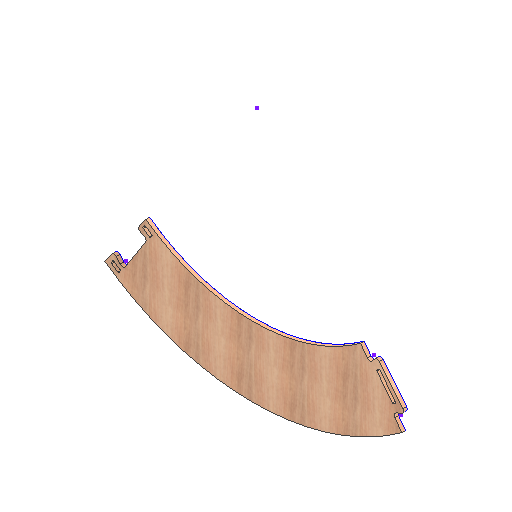
# Autodesk Inventor part: Platform C3
Saved by Autodesk Inventor 2021 (Build 250183000, 183)
## iProperties
Created: 2020-05-09
Part Number: Platform C3
Material: Wood (Birch)
Document SubType Name: Modeling
Designer: Dan Wikman
Density: 0.55 g/cm^3
Appearance: Birch - Natural Polished
Mass: 4368.22 g
Surface Area: 9555.55 cm^2
Volume: 7942.21 cm^3
Autodesk Inventor part; units mm, degrees
ref_plane "YZ Plane" through (0, 0, 0) normal (1, 0, 0) x (0, 1, 0)
ref_plane "XZ Plane" through (0, 0, 0) normal (0, 1, 0) x (-1, 0, 0)
ref_plane "XY Plane" through (0, 0, 0) normal (0, 0, 1) x (1, 0, 0)
sketch "CONTOURS" plane through (0, 0, 0) normal (0, 0, 1) x (1, 0, 0)
  line L0 (1187.1814, 538.0239) -> (1154.7956, 493.4487)
  arc A0 (1154.7956, 493.4487) -> (1161.7152, 471.2473) centre (1166.5264, 484.9258) ccw
  line L1 (1161.7152, 471.2473) -> (1177.6489, 465.6429)
  arc A1 (1185.5445, 442.6399) -> (1177.6489, 465.6429) centre (1172.5058, 451.021) ccw
  line L2 (1185.5445, 442.6399) -> (1088.242, 291.2628)
  arc A2 (1063.4384, 289.5524) -> (1088.242, 291.2628) centre (1075.2033, 299.6438) ccw
  line L3 (1063.4384, 289.5524) -> (1044.645, 311.4625)
  arc A3 (1044.645, 311.4625) -> (1021.9083, 310.545) centre (1033.6391, 302.0221) ccw
  line L4 (1021.9083, 310.545) -> (988.51, 264.5762)
  arc A4 (988.51, 264.5762) -> (2420.2584, 264.576) centre (1704.3843, 1251.0758) ccw
  line L5 (2420.2584, 264.576) -> (2386.86, 310.545)
  arc A5 (2393.4378, 333.9632) -> (2386.86, 310.545) centre (2399.3997, 319.6557) ccw
  line L6 (2393.4378, 333.9632) -> (2420.083, 345.0663)
  arc A6 (2420.083, 345.0663) -> (2425.7316, 367.6284) centre (2414.5057, 358.4507) ccw
  line L7 (2425.7316, 367.6284) -> (2311.8314, 506.9467)
  arc A7 (2311.8314, 506.9467) -> (2289.0833, 506.5717) centre (2300.6056, 497.769) ccw
  line L8 (2289.0833, 506.5717) -> (2278.8294, 493.1497)
  arc A8 (2253.9726, 493.4487) -> (2278.8294, 493.1497) centre (2266.5124, 502.5594) ccw
  line L9 (2253.9726, 493.4487) -> (2221.5869, 538.0239)
  arc A9 (1187.1814, 538.0239) -> (2221.5869, 538.0239) centre (1704.3841, 1250.9821) ccw
  constraints: 20 end point, 20 point on circle, 10 centre point
sketch "HOLES" plane through (0, 0, 0) normal (0, 0, 1) x (1, 0, 0)
  arc A0 (1185.5871, 509.2559) -> (1180.0259, 508.2196) centre (1183.3247, 505.9572) ccw
  line L0 (1185.5871, 509.2559) -> (1215.2756, 488.8945)
  arc A1 (1216.312, 483.3334) -> (1215.2756, 488.8945) centre (1213.0133, 485.5957) ccw
  line L1 (1216.312, 483.3334) -> (1210.0905, 474.2619)
  arc A2 (1204.5293, 473.2255) -> (1210.0905, 474.2619) centre (1206.7917, 476.5242) ccw
  line L2 (1204.5293, 473.2255) -> (1174.8407, 493.5869)
  arc A3 (1173.8044, 499.148) -> (1174.8407, 493.5869) centre (1177.1031, 496.8857) ccw
  line L3 (2383.598, 366.9908) -> (2380.4297, 364.5491)
  arc A4 (2374.8197, 365.2756) -> (2380.4297, 364.5491) centre (2377.988, 367.7173) ccw
  line L4 (2374.8197, 365.2756) -> (2300.3458, 461.907)
  arc A5 (2301.0723, 467.5171) -> (2300.3458, 461.907) centre (2303.5141, 464.3488) ccw
  line L5 (2301.0723, 467.5171) -> (2309.785, 474.2319)
  arc A6 (2315.395, 473.5054) -> (2309.785, 474.2319) centre (2312.2268, 471.0637) ccw
  line L6 (2315.395, 473.5054) -> (2389.8689, 376.874)
  arc A7 (2389.1424, 371.2639) -> (2389.8689, 376.874) centre (2386.7006, 374.4322) ccw
  line L7 (2389.1424, 371.2639) -> (2383.598, 366.9908)
  line L8 (1063.375, 260.339) -> (1057.1535, 251.2675)
  arc A8 (1051.5924, 250.2312) -> (1057.1535, 251.2675) centre (1053.8548, 253.5299) ccw
  line L9 (1051.5924, 250.2312) -> (1021.9038, 270.5926)
  arc A9 (1020.8674, 276.1537) -> (1021.9038, 270.5926) centre (1024.1662, 273.8913) ccw
  line L10 (1020.8674, 276.1537) -> (1027.089, 285.2252)
  arc A10 (1032.6501, 286.2616) -> (1027.089, 285.2252) centre (1030.3877, 282.9628) ccw
  line L11 (1032.6501, 286.2616) -> (1062.3387, 265.9002)
  arc A11 (1063.375, 260.339) -> (1062.3387, 265.9002) centre (1060.0763, 262.6014) ccw
  line L12 (1173.8044, 499.148) -> (1180.0259, 508.2196)
  constraints: 26 end point, 24 point on circle, 12 centre point
sketch "LETTERS" plane through (0, 0, 0) normal (0, 0, 1) x (1, 0, 0)
  line L0 (1208.7696, 324.759) -> (1209.0033, 324.7372)
  line L1 (1209.0033, 324.7372) -> (1209.2368, 324.7098)
  line L2 (1209.2368, 324.7098) -> (1209.4699, 324.6767)
  line L3 (1209.4699, 324.6767) -> (1209.7026, 324.638)
  line L4 (1209.7026, 324.638) -> (1209.9347, 324.5939)
  line L5 (1209.9347, 324.5939) -> (1210.166, 324.5444)
  line L6 (1210.166, 324.5444) -> (1210.3965, 324.4896)
  line L7 (1210.3965, 324.4896) -> (1210.6261, 324.4296)
  line L8 (1210.6261, 324.4296) -> (1210.8547, 324.3644)
  line L9 (1210.8547, 324.3644) -> (1211.082, 324.294)
  line L10 (1211.082, 324.294) -> (1211.3081, 324.2187)
  line L11 (1211.3081, 324.2187) -> (1211.5327, 324.1384)
  line L12 (1211.5327, 324.1384) -> (1211.7559, 324.0533)
  line L13 (1211.7559, 324.0533) -> (1211.9774, 323.9634)
  line L14 (1211.9774, 323.9634) -> (1212.1971, 323.8687)
  line L15 (1212.1971, 323.8687) -> (1212.415, 323.7694)
  line L16 (1212.415, 323.7694) -> (1212.6308, 323.6655)
  line L17 (1212.6308, 323.6655) -> (1212.8446, 323.5572)
  line L18 (1212.8446, 323.5572) -> (1213.0562, 323.4444)
  line L19 (1213.0562, 323.4444) -> (1213.2655, 323.3273)
  line L20 (1213.2655, 323.3273) -> (1213.4724, 323.2058)
  line L21 (1213.4724, 323.2058) -> (1213.6769, 323.0802)
  line L22 (1213.6769, 323.0802) -> (1213.8789, 322.9504)
  line L23 (1213.8789, 322.9504) -> (1214.0783, 322.8166)
  line L24 (1214.0783, 322.8166) -> (1214.275, 322.6787)
  line L25 (1214.275, 322.6787) -> (1214.469, 322.5369)
  line L26 (1214.469, 322.5369) -> (1214.6601, 322.3913)
  line L27 (1214.6601, 322.3913) -> (1214.8483, 322.2419)
  line L28 (1214.8483, 322.2419) -> (1215.0335, 322.0887)
  line L29 (1215.0335, 322.0887) -> (1215.2156, 321.9319)
  line L30 (1215.2156, 321.9319) -> (1215.3946, 321.7715)
  line L31 (1215.3946, 321.7715) -> (1215.5703, 321.6076)
  line L32 (1215.5703, 321.6076) -> (1215.7426, 321.4402)
  line L33 (1215.7426, 321.4402) -> (1215.9116, 321.2695)
  line L34 (1215.9116, 321.2695) -> (1216.0771, 321.0955)
  line L35 (1216.0771, 321.0955) -> (1216.2389, 320.9182)
  line L36 (1216.2389, 320.9182) -> (1216.3972, 320.7378)
  line L37 (1216.3972, 320.7378) -> (1216.5517, 320.5543)
  line L38 (1216.5517, 320.5543) -> (1216.7024, 320.3678)
  line L39 (1216.7024, 320.3678) -> (1216.8491, 320.1783)
  line L40 (1216.8491, 320.1783) -> (1216.9919, 319.9859)
  line L41 (1216.9919, 319.9859) -> (1217.1307, 319.7908)
  line L42 (1217.1307, 319.7908) -> (1217.2653, 319.5929)
  line L43 (1217.2653, 319.5929) -> (1217.3956, 319.3923)
  line L44 (1217.3956, 319.3923) -> (1217.5217, 319.1891)
  line L45 (1217.5217, 319.1891) -> (1217.6434, 318.9834)
  line L46 (1217.6434, 318.9834) -> (1217.7606, 318.7752)
  line L47 (1217.7606, 318.7752) -> (1217.8733, 318.5647)
  line L48 (1217.8733, 318.5647) -> (1217.9813, 318.3518)
  line L49 (1217.9813, 318.3518) -> (1218.0846, 318.1367)
  line L50 (1218.0846, 318.1367) -> (1218.1832, 317.9195)
  line L51 (1218.1832, 317.9195) -> (1218.2769, 317.7002)
  line L52 (1218.2769, 317.7002) -> (1218.3657, 317.4791)
  line L53 (1218.3657, 317.4791) -> (1218.4496, 317.2562)
  line L54 (1218.4496, 317.2562) -> (1218.5286, 317.0317)
  line L55 (1218.5286, 317.0317) -> (1218.6024, 316.8056)
  line L56 (1218.6024, 316.8056) -> (1218.6712, 316.5781)
  line L57 (1218.6712, 316.5781) -> (1218.7348, 316.3494)
  line L58 (1218.7348, 316.3494) -> (1218.7932, 316.1195)
  line L59 (1218.7932, 316.1195) -> (1218.8464, 315.8885)
  line L60 (1218.8464, 315.8885) -> (1218.8942, 315.6566)
  line L61 (1218.8942, 315.6566) -> (1218.9366, 315.424)
  line L62 (1218.9366, 315.424) -> (1218.9736, 315.1906)
  line L63 (1218.9736, 315.1906) -> (1219.0051, 314.9567)
  line L64 (1219.0051, 314.9567) -> (1219.031, 314.7224)
  line L65 (1219.031, 314.7224) -> (1219.0514, 314.4877)
  line L66 (1219.0514, 314.4877) -> (1219.0661, 314.2529)
  line L67 (1219.0661, 314.2529) -> (1219.0751, 314.0179)
  line L68 (1219.0751, 314.0179) -> (1219.0783, 313.783)
  line L69 (1219.0783, 313.783) -> (1219.0757, 313.5483)
  line L70 (1219.0757, 313.5483) -> (1219.0672, 313.3139)
  line L71 (1219.0672, 313.3139) -> (1219.0528, 313.0799)
  line L72 (1219.0528, 313.0799) -> (1219.0324, 312.8464)
  line L73 (1219.0324, 312.8464) -> (1219.0059, 312.6136)
  line L74 (1219.0059, 312.6136) -> (1218.9733, 312.3815)
  line L75 (1218.9733, 312.3815) -> (1218.9346, 312.1503)
  line L76 (1218.9346, 312.1503) -> (1218.8897, 311.9202)
  line L77 (1218.8897, 311.9202) -> (1218.8385, 311.6911)
  line L78 (1218.8385, 311.6911) -> (1218.7809, 311.4634)
  line L79 (1218.7809, 311.4634) -> (1218.717, 311.237)
  line L80 (1218.717, 311.237) -> (1218.6466, 311.0121)
  line L81 (1218.6466, 311.0121) -> (1218.5698, 310.7888)
  line L82 (1218.5698, 310.7888) -> (1218.4866, 310.5673)
  line L83 (1218.4866, 310.5673) -> (1218.3972, 310.3477)
  line L84 (1218.3972, 310.3477) -> (1218.3016, 310.1302)
  line L85 (1218.3016, 310.1302) -> (1218.2, 309.9149)
  line L86 (1218.2, 309.9149) -> (1218.0925, 309.7021)
  line L87 (1218.0925, 309.7021) -> (1217.9793, 309.4917)
  line L88 (1217.9793, 309.4917) -> (1217.8604, 309.2841)
  line L89 (1217.8604, 309.2841) -> (1217.7359, 309.0793)
  line L90 (1217.7359, 309.0793) -> (1217.6061, 308.8776)
  line L91 (1217.6061, 308.8776) -> (1217.471, 308.679)
  line L92 (1217.471, 308.679) -> (1217.3307, 308.4837)
  line L93 (1217.3307, 308.4837) -> (1217.1853, 308.2919)
  line L94 (1217.1853, 308.2919) -> (1217.035, 308.1038)
  line L95 (1217.035, 308.1038) -> (1216.8799, 307.9194)
  line L96 (1216.8799, 307.9194) -> (1216.7202, 307.739)
  line L97 (1216.7202, 307.739) -> (1216.5558, 307.5626)
  line L98 (1216.5558, 307.5626) -> (1216.3871, 307.3906)
  line L99 (1216.3871, 307.3906) -> (1216.214, 307.2229)
  line L100 (1216.214, 307.2229) -> (1216.0366, 307.0598)
  line L101 (1216.0366, 307.0598) -> (1215.8552, 306.9014)
  line L102 (1215.8552, 306.9014) -> (1215.6699, 306.7478)
  line L103 (1215.6699, 306.7478) -> (1215.4807, 306.5993)
  line L104 (1215.4807, 306.5993) -> (1215.2878, 306.456)
  line L105 (1215.2878, 306.456) -> (1215.0912, 306.318)
  line L106 (1215.0912, 306.318) -> (1214.8912, 306.1855)
  line L107 (1214.8912, 306.1855) -> (1214.6878, 306.0587)
  line L108 (1214.6878, 306.0587) -> (1214.4812, 305.9377)
  line L109 (1214.4812, 305.9377) -> (1214.2715, 305.8226)
  line L110 (1214.2715, 305.8226) -> (1214.0588, 305.7136)
  line L111 (1214.0588, 305.7136) -> (1213.8431, 305.6109)
  line L112 (1213.8431, 305.6109) -> (1213.6248, 305.5146)
  line L113 (1213.6248, 305.5146) -> (1213.4038, 305.4249)
  line L114 (1213.4038, 305.4249) -> (1213.1803, 305.3417)
  line L115 (1213.1803, 305.3417) -> (1212.9546, 305.2653)
  line L116 (1212.9546, 305.2653) -> (1212.7269, 305.1955)
  line L117 (1212.7269, 305.1955) -> (1212.4974, 305.1324)
  line L118 (1212.4974, 305.1324) -> (1212.2662, 305.0761)
  line L119 (1212.2662, 305.0761) -> (1212.0336, 305.0266)
  line L120 (1212.0336, 305.0266) -> (1211.7997, 304.984)
  line L121 (1211.7997, 304.984) -> (1211.5648, 304.9482)
  line L122 (1211.5648, 304.9482) -> (1211.3291, 304.9193)
  line L123 (1211.3291, 304.9193) -> (1211.0928, 304.8974)
  line L124 (1211.0928, 304.8974) -> (1210.856, 304.8825)
  line L125 (1210.856, 304.8825) -> (1210.6191, 304.8745)
  line L126 (1210.6191, 304.8745) -> (1210.382, 304.8736)
  line L127 (1210.382, 304.8736) -> (1210.1452, 304.8798)
  line L128 (1210.1452, 304.8798) -> (1209.9088, 304.8931)
  line L129 (1209.9088, 304.8931) -> (1209.6729, 304.9136)
  line L130 (1209.6729, 304.9136) -> (1209.4378, 304.9413)
  line L131 (1209.4378, 304.9413) -> (1209.2037, 304.9762)
  line L132 (1209.2037, 304.9762) -> (1208.9708, 305.0183)
  line L133 (1208.9708, 305.0183) -> (1208.7392, 305.0678)
  line L134 (1208.7392, 305.0678) -> (1208.5093, 305.1246)
  line L135 (1208.5093, 305.1246) -> (1208.2811, 305.1888)
  line L136 (1208.2811, 305.1888) -> (1208.0549, 305.2604)
  line L137 (1208.0549, 305.2604) -> (1207.831, 305.3394)
  line L138 (1207.831, 305.3394) -> (1207.6094, 305.4259)
  line L139 (1207.6094, 305.4259) -> (1207.3904, 305.52)
  line L140 (1207.3904, 305.52) -> (1207.1741, 305.6215)
  line L141 (1207.1741, 305.6215) -> (1206.9609, 305.7306)
  line L142 (1206.9609, 305.7306) -> (1206.7508, 305.8474)
  line L143 (1206.7508, 305.8474) -> (1206.5442, 305.9718)
  line L144 (1206.5442, 305.9718) -> (1206.4422, 306.0369)
  line L145 (1206.4422, 306.0369) -> (1206.3411, 306.1039)
  line L146 (1200.6132, 311.8395) -> (1200.4954, 312.0474)
  line L147 (1200.4954, 312.0474) -> (1200.3834, 312.2585)
  line L148 (1200.3834, 312.2585) -> (1200.2774, 312.4725)
  line L149 (1200.2774, 312.4725) -> (1200.1773, 312.6893)
  line L150 (1200.1773, 312.6893) -> (1200.0833, 312.9088)
  line L151 (1200.0833, 312.9088) -> (1199.9953, 313.1306)
  line L152 (1199.9953, 313.1306) -> (1199.9133, 313.3547)
  line L153 (1199.9133, 313.3547) -> (1199.8375, 313.5809)
  line L154 (1199.8375, 313.5809) -> (1199.7678, 313.809)
  line L155 (1199.7678, 313.809) -> (1199.7043, 314.0389)
  line L156 (1199.7043, 314.0389) -> (1199.647, 314.2703)
  line L157 (1199.647, 314.2703) -> (1199.596, 314.5031)
  line L158 (1199.596, 314.5031) -> (1199.5512, 314.7371)
  line L159 (1199.5512, 314.7371) -> (1199.5127, 314.9721)
  line L160 (1199.5127, 314.9721) -> (1199.4806, 315.208)
  line L161 (1199.4806, 315.208) -> (1199.4549, 315.4446)
  line L162 (1199.4549, 315.4446) -> (1199.4356, 315.6817)
  line L163 (1199.4356, 315.6817) -> (1199.4228, 315.9191)
  line L164 (1199.4228, 315.9191) -> (1199.4164, 316.1567)
  line L165 (1199.4164, 316.1567) -> (1199.4166, 316.3943)
  line L166 (1199.4166, 316.3943) -> (1199.4234, 316.6317)
  line L167 (1199.4234, 316.6317) -> (1199.4367, 316.8687)
  line L168 (1199.4367, 316.8687) -> (1199.4567, 317.1052)
  line L169 (1199.4567, 317.1052) -> (1199.4833, 317.341)
  line L170 (1199.4833, 317.341) -> (1199.5167, 317.5759)
  line L171 (1199.5167, 317.5759) -> (1199.5568, 317.8098)
  line L172 (1199.5568, 317.8098) -> (1199.6036, 318.0424)
  line L173 (1199.6036, 318.0424) -> (1199.6573, 318.2736)
  line L174 (1199.6573, 318.2736) -> (1199.7178, 318.5032)
  line L175 (1199.7178, 318.5032) -> (1199.7852, 318.731)
  line L176 (1199.7852, 318.731) -> (1199.8595, 318.9569)
  line L177 (1199.8595, 318.9569) -> (1199.9408, 319.1808)
  line L178 (1199.9408, 319.1808) -> (1200.029, 319.4023)
  line L179 (1200.029, 319.4023) -> (1200.124, 319.6214)
  line L180 (1200.124, 319.6214) -> (1200.2257, 319.8379)
  line L181 (1200.2257, 319.8379) -> (1200.3338, 320.0517)
  line L182 (1200.3338, 320.0517) -> (1200.4483, 320.2627)
  line L183 (1200.4483, 320.2627) -> (1200.5689, 320.4706)
  line L184 (1200.5689, 320.4706) -> (1200.6955, 320.6754)
  line L185 (1200.6955, 320.6754) -> (1200.8279, 320.8769)
  line L186 (1200.8279, 320.8769) -> (1200.966, 321.075)
  line L187 (1200.966, 321.075) -> (1201.1095, 321.2695)
  line L188 (1201.1095, 321.2695) -> (1201.2584, 321.4603)
  line L189 (1201.2584, 321.4603) -> (1201.4123, 321.6472)
  line L190 (1201.4123, 321.6472) -> (1201.5713, 321.8301)
  line L191 (1201.5713, 321.8301) -> (1201.7351, 322.0088)
  line L192 (1201.7351, 322.0088) -> (1201.9035, 322.1833)
  line L193 (1201.9035, 322.1833) -> (1202.0764, 322.3533)
  line L194 (1202.0764, 322.3533) -> (1202.2535, 322.5187)
  line L195 (1202.2535, 322.5187) -> (1202.4349, 322.6794)
  line L196 (1202.4349, 322.6794) -> (1202.6202, 322.8352)
  line L197 (1202.6202, 322.8352) -> (1202.8093, 322.986)
  line L198 (1202.8093, 322.986) -> (1203.002, 323.1317)
  line L199 (1203.002, 323.1317) -> (1203.1982, 323.272)
  line L200 (1203.1982, 323.272) -> (1203.3977, 323.4069)
  line L201 (1203.3977, 323.4069) -> (1203.6004, 323.5362)
  line L202 (1203.6004, 323.5362) -> (1203.806, 323.6598)
  line L203 (1203.806, 323.6598) -> (1204.0144, 323.7774)
  line L204 (1204.0144, 323.7774) -> (1204.2254, 323.8891)
  line L205 (1204.2254, 323.8891) -> (1204.4389, 323.9946)
  line L206 (1204.4389, 323.9946) -> (1204.6547, 324.0938)
  line L207 (1204.6547, 324.0938) -> (1204.8726, 324.1865)
  line L208 (1204.8726, 324.1865) -> (1205.0925, 324.2727)
  line L209 (1205.0925, 324.2727) -> (1205.3142, 324.352)
  line L210 (1205.3142, 324.352) -> (1205.5375, 324.4246)
  line L211 (1205.5375, 324.4246) -> (1205.7624, 324.4903)
  line L212 (1205.7624, 324.4903) -> (1205.9886, 324.5493)
  line L213 (1205.9886, 324.5493) -> (1206.2161, 324.6016)
  line L214 (1206.2161, 324.6016) -> (1206.4448, 324.6474)
  line L215 (1206.4448, 324.6474) -> (1206.6745, 324.6866)
  line L216 (1206.6745, 324.6866) -> (1206.9051, 324.7194)
  line L217 (1206.9051, 324.7194) -> (1207.1366, 324.7459)
  line L218 (1207.1366, 324.7459) -> (1207.3687, 324.766)
  line L219 (1208.5357, 324.775) -> (1208.7696, 324.759)
  line L220 (1207.6014, 324.7799) -> (1207.8346, 324.7877)
  line L221 (1207.8346, 324.7877) -> (1208.0681, 324.7895)
  line L222 (1208.0681, 324.7895) -> (1208.3019, 324.7852)
  line L223 (1208.3019, 324.7852) -> (1208.5357, 324.775)
  line L224 (1207.3687, 324.766) -> (1207.6014, 324.7799)
  constraints: 450 end point, 5 perpendicular
extrude "Extrusion2" add sketch "CONTOURS" along normal blind 18
extrude "Extrusion3" cut sketch "HOLES" along normal blind 18
body "Solid1"
